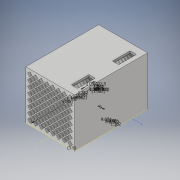
# Autodesk Inventor part: Double Holder V1
Saved by Autodesk Inventor 2019 (Build 230136000, 136)
## iProperties
Created: 2018-11-20
Part Number: Double Holder V1
Material: Generic
Document SubType Name: Modeling
Designer: Ashley
Density: 1 g/cm^3
Appearance: Default
Author: Ashley
Autodesk Inventor part; units mm, degrees
(part 1 of 2)
ref_plane "YZ Plane" through (0, 0, 0) normal (1, 0, 0) x (0, 1, 0)
ref_plane "XZ Plane" through (0, 0, 0) normal (0, 1, 0) x (-1, 0, 0)
ref_plane "XY Plane" through (0, 0, 0) normal (0, 0, 1) x (1, 0, 0)
sketch "Main Body Sketch" plane through (0, 0, 0) normal (0, 1, 0) x (-1, 0, 0)
  line L0 (-38.5, 7.5) -> (38.5, 7.5)
  line L1 (38.5, 7.5) -> (38.5, 57.5)
  line L2 (38.5, 57.5) -> (-38.5, 57.5)
  line L3 (-38.5, 57.5) -> (-38.5, 7.5)
  line L4 (0, 222.8068) -> (0, -187.3036) construction
  line L5 (63.0186, 0) -> (-52.8672, 0) construction
  line L6 (-38.5, -7.5) -> (38.5, -7.5)
  line L7 (38.5, -7.5) -> (38.5, -57.5)
  line L8 (38.5, -57.5) -> (-38.5, -57.5)
  line L9 (-38.5, -57.5) -> (-38.5, -7.5)
  line L10 (0, -222.8068) -> (0, 187.3036) construction
  point P0 (0, 0)
  dimension "d2" = 50
  dimension "d3" = 77
  dimension "d4" = 38.5
  dimension "d5" = 38.5
  dimension "d6" = 7.5
  constraints: 22 end point, 6 symmetric about line, 3 horizontal, 2 parallel, 2 vertical, 1 perpendicular
  measures "d2" distance of L0.end L1.end
  measures "d3" distance of L1.end L2.end
  measures "d4" distance between parallel lines of L4 L1
  measures "d5" distance between parallel lines of L3 L4
  measures "d6" distance between parallel lines of L5 L0
extrude "Main Body Extrusion" add sketch "Main Body Sketch" along normal blind 77
sketch "Main Compartments Sketch" plane through (-38.5, 0, 7.5) normal (-1, 0, 0) x (0, 0, 1)
  line L0 (0, 0) -> (50, 0) construction
  line L1 (-61.5, 3.5) -> (-18.5, 3.5)
  line L2 (-18.5, 3.5) -> (-18.5, 73.5)
  line L3 (-18.5, 73.5) -> (-61.5, 73.5)
  line L4 (-61.5, 73.5) -> (-61.5, 3.5)
  line L5 (-65, 77) -> (-15, 77) construction
  line L6 (-15, 0) -> (-65, 0) construction
  line L7 (-65, 0) -> (-65, 77) construction
  line L8 (-15, 0) -> (-15, 77) construction
  line L9 (-7.5, -40.8537) -> (-7.5, 113.2873) construction
  line L10 (46.5, 3.5) -> (3.5, 3.5)
  line L11 (3.5, 3.5) -> (3.5, 73.5)
  line L12 (3.5, 73.5) -> (46.5, 73.5)
  line L13 (46.5, 73.5) -> (46.5, 3.5)
  line L14 (50, 77) -> (0, 77) construction
  line L15 (0, 0) -> (50, 0) construction
  line L16 (50, 0) -> (50, 77) construction
  line L17 (0, 0) -> (0, 77) construction
  point P0 (-7.5, 0)
  dimension "d10" = 70
  dimension "d11" = 3.5
  dimension "d12" = 3.5
  dimension "d13" = 43
  dimension "d14" = 3.5
  dimension "d15" = 3.5
  dimension "d16" = 3.5
  dimension "d17" = 3.5
  constraints: 26 end point, 4 symmetric about line, 2 parallel, 2 vertical, 1 horizontal, 1 perpendicular
  measures "d10" distance of L3.end L1.start
  measures "d11" distance between parallel lines of L5 L3
  measures "d12" distance between parallel lines of L6 L1
  measures "d13" distance between parallel lines of L2 L4
  measures "d14" distance between parallel lines of L7 L4
  measures "d15" distance between parallel lines of L8 L2
  measures "d16" distance between parallel lines of L17 L11
  measures "d17" distance between parallel lines of L0 L10
extrude "Main Compartments Extrusion" cut sketch "Main Compartments Sketch" against normal blind 73.5
sketch "Tape Measure Hole Sketch" plane through (0, 77, 0) normal (0, 1, 0) x (1, 0, 0)
  line L0 (38.5, -57.5) -> (38.5, 57.5) construction
  line L1 (22, -46.5) -> (32, -46.5)
  line L2 (32, -46.5) -> (32, -18.5)
  line L3 (32, -18.5) -> (22, -18.5)
  line L4 (22, -18.5) -> (22, -46.5)
  line L5 (-52.0293, 0) -> (49.471, 0) construction
  line L6 (-38.5, -11) -> (35, -11) construction
  line L7 (4.7749, -11) -> (35, -11) construction
  line L8 (-38.5, -54) -> (35, -54) construction
  line L9 (22, 46.5) -> (32, 46.5)
  line L10 (32, 46.5) -> (32, 18.5)
  line L11 (32, 18.5) -> (22, 18.5)
  line L12 (22, 18.5) -> (22, 46.5)
  line L13 (-38.5, -54) -> (35, -54) construction
  line L14 (35, -54) -> (35, -11) construction
  point P0 (0, 0)
  dimension "d26" = 10
  dimension "d27" = 6.5
  dimension "d28" = 28
  dimension "d32" = 11
  dimension "d33" = 43
  dimension "d34" = 7.5
  dimension "d35" = 7.5
  dimension "d38" = 3.5
  dimension "d39" = 3
  constraints: 22 end point, 4 horizontal, 4 symmetric about line, 3 parallel, 1 collinear, 1 perpendicular, 1 point on line, 1 vertical
  measures "d26" distance of L2.end L3.end
  measures "d27" distance between parallel lines of L0 L2
  measures "d28" distance of L3.end L1.start
  measures "d32" distance between parallel lines of L5 L6
  measures "d33" distance between parallel lines of L6 L8
  measures "d34" distance between parallel lines of L8 L1
  measures "d35" distance between parallel lines of L3 L7
  measures "d38" distance between parallel lines of L0 L14
  measures "d39" distance between parallel lines of L14 L2
extrude "Tape Measure Holes Cut" cut sketch "Tape Measure Hole Sketch" against normal up to surface (3.5 mm away)
fillet "Tape Measure Holes Softening" radius 1 8 edges at (22, 75.25, 46.5) (32, 75.25, 46.5) (22, 75.25, 18.5) (32, 75.25, 18.5) (32, 75.25, -46.5) (22, 75.25, -46.5) (22, 75.25, -18.5) (32, 75.25, -18.5)
sketch "Center Sketch" plane through (38.5, 0, 7.5) normal (0, 0, -1) x (-1, 0, 0)
  line L0 (77, 77) -> (0, 77)
  line L1 (0, 77) -> (0, 0)
  line L2 (0, 0) -> (77, 0)
  line L3 (77, 0) -> (77, 77)
  point P0 (38.5, 0)
  constraints: 8 end point, 2 parallel, 1 horizontal, 1 perpendicular
extrude "Center Extrusion" add sketch "Center Sketch" along normal up to surface (15 mm away)
sketch "Swiss Holes Sketch" plane through (38.5, 0, -57.5) normal (0, 0, -1) x (-1, 0, 0)
  line L0 (0, 77) -> (77, 77) construction
  line L1 (77, 73.5) -> (3.5, 73.5) construction
  line L2 (3.5, 73.5) -> (3.5, 3.5) construction
  line L3 (77, 73.5) -> (3.5, 73.5) construction
  line L4 (3.5, 73.5) -> (3.5, 3.5) construction
  line L5 (3.5, 3.5) -> (77, 3.5) construction
  line L6 (66.9969, 69.9645) -> (70.5325, 73.5)
  line L7 (70.5325, 73.5) -> (74.068, 69.9645)
  line L8 (74.068, 69.9645) -> (70.5325, 66.4289)
  line L9 (70.5325, 66.4289) -> (66.9969, 69.9645)
  line L10 (77, 0) -> (77, 77) construction
  line L11 (61.4615, 66.4289) -> (57.9259, 69.9645)
  line L12 (61.4615, 73.5) -> (64.997, 69.9645)
  line L13 (64.997, 69.9645) -> (61.4615, 66.4289)
  line L14 (67.929, 73.5) -> (-5.571, 73.5) construction
  line L15 (57.9259, 69.9645) -> (61.4615, 73.5)
  line L16 (52.3905, 66.4289) -> (48.8549, 69.9645)
  line L17 (52.3905, 73.5) -> (55.926, 69.9645)
  line L18 (55.926, 69.9645) -> (52.3905, 66.4289)
  line L19 (58.858, 73.5) -> (-14.642, 73.5) construction
  line L20 (48.8549, 69.9645) -> (52.3905, 73.5)
  line L21 (43.3195, 66.4289) -> (39.7839, 69.9645)
  line L22 (43.3195, 73.5) -> (46.855, 69.9645)
  line L23 (46.855, 69.9645) -> (43.3195, 66.4289)
  line L24 (49.787, 73.5) -> (-23.713, 73.5) construction
  line L25 (39.7839, 69.9645) -> (43.3195, 73.5)
  line L26 (34.2485, 66.4289) -> (30.7129, 69.9645)
  line L27 (34.2485, 73.5) -> (37.784, 69.9645)
  line L28 (37.784, 69.9645) -> (34.2485, 66.4289)
  line L29 (40.716, 73.5) -> (-32.784, 73.5) construction
  line L30 (30.7129, 69.9645) -> (34.2485, 73.5)
  line L31 (25.1775, 66.4289) -> (21.6419, 69.9645)
  line L32 (25.1775, 73.5) -> (28.713, 69.9645)
  line L33 (28.713, 69.9645) -> (25.1775, 66.4289)
  line L34 (31.645, 73.5) -> (-41.855, 73.5) construction
  line L35 (21.6419, 69.9645) -> (25.1775, 73.5)
  line L36 (16.1065, 66.4289) -> (12.5709, 69.9645)
  line L37 (16.1065, 73.5) -> (19.642, 69.9645)
  line L38 (19.642, 69.9645) -> (16.1065, 66.4289)
  line L39 (22.574, 73.5) -> (-50.926, 73.5) construction
  line L40 (12.5709, 69.9645) -> (16.1065, 73.5)
  line L41 (7.0355, 66.4289) -> (3.4999, 69.9645)
  line L42 (7.0355, 73.5) -> (10.571, 69.9645)
  line L43 (10.571, 69.9645) -> (7.0355, 66.4289)
  line L44 (13.503, 73.5) -> (-59.997, 73.5) construction
  line L45 (3.4999, 69.9645) -> (7.0355, 73.5)
  line L46 (70.5325, 57.4489) -> (66.9969, 60.9845)
  line L47 (70.5325, 64.52) -> (74.068, 60.9845)
  line L48 (74.068, 60.9845) -> (70.5325, 57.4489)
  line L49 (77, 64.52) -> (3.5, 64.52) construction
  line L50 (66.9969, 60.9845) -> (70.5325, 64.52)
  line L51 (61.4615, 57.4489) -> (57.9259, 60.9845)
  line L52 (61.4615, 64.52) -> (64.997, 60.9845)
  line L53 (64.997, 60.9845) -> (61.4615, 57.4489)
  line L54 (67.929, 64.52) -> (-5.571, 64.52) construction
  line L55 (57.9259, 60.9845) -> (61.4615, 64.52)
  line L56 (52.3905, 57.4489) -> (48.8549, 60.9845)
  line L57 (52.3905, 64.52) -> (55.926, 60.9845)
  line L58 (55.926, 60.9845) -> (52.3905, 57.4489)
  line L59 (58.858, 64.52) -> (-14.642, 64.52) construction
  line L60 (48.8549, 60.9845) -> (52.3905, 64.52)
  line L61 (43.3195, 57.4489) -> (39.7839, 60.9845)
  line L62 (43.3195, 64.52) -> (46.855, 60.9845)
  line L63 (46.855, 60.9845) -> (43.3195, 57.4489)
  line L64 (49.787, 64.52) -> (-23.713, 64.52) construction
  line L65 (39.7839, 60.9845) -> (43.3195, 64.52)
  line L66 (34.2485, 57.4489) -> (30.7129, 60.9845)
  line L67 (34.2485, 64.52) -> (37.784, 60.9845)
  line L68 (37.784, 60.9845) -> (34.2485, 57.4489)
  line L69 (40.716, 64.52) -> (-32.784, 64.52) construction
  line L70 (30.7129, 60.9845) -> (34.2485, 64.52)
  line L71 (25.1775, 57.4489) -> (21.6419, 60.9845)
  line L72 (25.1775, 64.52) -> (28.713, 60.9845)
  line L73 (28.713, 60.9845) -> (25.1775, 57.4489)
  line L74 (31.645, 64.52) -> (-41.855, 64.52) construction
  line L75 (21.6419, 60.9845) -> (25.1775, 64.52)
  line L76 (16.1065, 57.4489) -> (12.5709, 60.9845)
  line L77 (16.1065, 64.52) -> (19.642, 60.9845)
  line L78 (19.642, 60.9845) -> (16.1065, 57.4489)
  line L79 (22.574, 64.52) -> (-50.926, 64.52) construction
  line L80 (12.5709, 60.9845) -> (16.1065, 64.52)
  line L81 (7.0355, 57.4489) -> (3.4999, 60.9845)
  line L82 (7.0355, 64.52) -> (10.571, 60.9845)
  line L83 (10.571, 60.9845) -> (7.0355, 57.4489)
  line L84 (13.503, 64.52) -> (-59.997, 64.52) construction
  line L85 (3.4999, 60.9845) -> (7.0355, 64.52)
  line L86 (70.5325, 48.4689) -> (66.9969, 52.0045)
  line L87 (70.5325, 55.54) -> (74.068, 52.0045)
  line L88 (74.068, 52.0045) -> (70.5325, 48.4689)
  line L89 (77, 55.54) -> (3.5, 55.54) construction
  line L90 (66.9969, 52.0045) -> (70.5325, 55.54)
  line L91 (61.4615, 48.4689) -> (57.9259, 52.0045)
  line L92 (61.4615, 55.54) -> (64.997, 52.0045)
  line L93 (64.997, 52.0045) -> (61.4615, 48.4689)
  line L94 (67.929, 55.54) -> (-5.571, 55.54) construction
  line L95 (57.9259, 52.0045) -> (61.4615, 55.54)
  line L96 (52.3905, 48.4689) -> (48.8549, 52.0045)
  line L97 (52.3905, 55.54) -> (55.926, 52.0045)
  line L98 (55.926, 52.0045) -> (52.3905, 48.4689)
  line L99 (58.858, 55.54) -> (-14.642, 55.54) construction
  line L100 (48.8549, 52.0045) -> (52.3905, 55.54)
  line L101 (43.3195, 48.4689) -> (39.7839, 52.0045)
  line L102 (43.3195, 55.54) -> (46.855, 52.0045)
  line L103 (46.855, 52.0045) -> (43.3195, 48.4689)
  line L104 (49.787, 55.54) -> (-23.713, 55.54) construction
  line L105 (39.7839, 52.0045) -> (43.3195, 55.54)
  line L106 (34.2485, 48.4689) -> (30.7129, 52.0045)
  line L107 (34.2485, 55.54) -> (37.784, 52.0045)
  line L108 (37.784, 52.0045) -> (34.2485, 48.4689)
  line L109 (40.716, 55.54) -> (-32.784, 55.54) construction
  line L110 (30.7129, 52.0045) -> (34.2485, 55.54)
  line L111 (25.1775, 48.4689) -> (21.6419, 52.0045)
  line L112 (25.1775, 55.54) -> (28.713, 52.0045)
  line L113 (28.713, 52.0045) -> (25.1775, 48.4689)
  line L114 (31.645, 55.54) -> (-41.855, 55.54) construction
  line L115 (21.6419, 52.0045) -> (25.1775, 55.54)
  line L116 (16.1065, 48.4689) -> (12.5709, 52.0045)
  line L117 (16.1065, 55.54) -> (19.642, 52.0045)
  line L118 (19.642, 52.0045) -> (16.1065, 48.4689)
  line L119 (22.574, 55.54) -> (-50.926, 55.54) construction
  line L120 (12.5709, 52.0045) -> (16.1065, 55.54)
  line L121 (7.0355, 48.4689) -> (3.4999, 52.0045)
  line L122 (7.0355, 55.54) -> (10.571, 52.0045)
  line L123 (10.571, 52.0045) -> (7.0355, 48.4689)
  line L124 (13.503, 55.54) -> (-59.997, 55.54) construction
  line L125 (3.4999, 52.0045) -> (7.0355, 55.54)
  line L126 (70.5325, 39.4889) -> (66.9969, 43.0245)
  line L127 (70.5325, 46.56) -> (74.068, 43.0245)
  line L128 (74.068, 43.0245) -> (70.5325, 39.4889)
  line L129 (77, 46.56) -> (3.5, 46.56) construction
  line L130 (66.9969, 43.0245) -> (70.5325, 46.56)
  line L131 (61.4615, 39.4889) -> (57.9259, 43.0245)
  line L132 (61.4615, 46.56) -> (64.997, 43.0245)
  line L133 (64.997, 43.0245) -> (61.4615, 39.4889)
  line L134 (67.929, 46.56) -> (-5.571, 46.56) construction
  line L135 (57.9259, 43.0245) -> (61.4615, 46.56)
  line L136 (52.3905, 39.4889) -> (48.8549, 43.0245)
  line L137 (52.3905, 46.56) -> (55.926, 43.0245)
  line L138 (55.926, 43.0245) -> (52.3905, 39.4889)
  line L139 (58.858, 46.56) -> (-14.642, 46.56) construction
  line L140 (48.8549, 43.0245) -> (52.3905, 46.56)
  line L141 (43.3195, 39.4889) -> (39.7839, 43.0245)
  line L142 (43.3195, 46.56) -> (46.855, 43.0245)
  line L143 (46.855, 43.0245) -> (43.3195, 39.4889)
  line L144 (49.787, 46.56) -> (-23.713, 46.56) construction
  line L145 (39.7839, 43.0245) -> (43.3195, 46.56)
  line L146 (34.2485, 39.4889) -> (30.7129, 43.0245)
  line L147 (34.2485, 46.56) -> (37.784, 43.0245)
  line L148 (37.784, 43.0245) -> (34.2485, 39.4889)
  line L149 (40.716, 46.56) -> (-32.784, 46.56) construction
  line L150 (30.7129, 43.0245) -> (34.2485, 46.56)
  line L151 (25.1775, 39.4889) -> (21.6419, 43.0245)
  line L152 (25.1775, 46.56) -> (28.713, 43.0245)
  line L153 (28.713, 43.0245) -> (25.1775, 39.4889)
  line L154 (31.645, 46.56) -> (-41.855, 46.56) construction
  line L155 (21.6419, 43.0245) -> (25.1775, 46.56)
  line L156 (16.1065, 39.4889) -> (12.5709, 43.0245)
  line L157 (16.1065, 46.56) -> (19.642, 43.0245)
  line L158 (19.642, 43.0245) -> (16.1065, 39.4889)
  line L159 (22.574, 46.56) -> (-50.926, 46.56) construction
  line L160 (12.5709, 43.0245) -> (16.1065, 46.56)
  line L161 (7.0355, 39.4889) -> (3.4999, 43.0245)
  line L162 (7.0355, 46.56) -> (10.571, 43.0245)
  line L163 (10.571, 43.0245) -> (7.0355, 39.4889)
  line L164 (13.503, 46.56) -> (-59.997, 46.56) construction
  line L165 (3.4999, 43.0245) -> (7.0355, 46.56)
  line L166 (70.5325, 30.5089) -> (66.9969, 34.0445)
  line L167 (70.5325, 37.58) -> (74.068, 34.0445)
  line L168 (74.068, 34.0445) -> (70.5325, 30.5089)
  line L169 (77, 37.58) -> (3.5, 37.58) construction
  line L170 (66.9969, 34.0445) -> (70.5325, 37.58)
  line L171 (61.4615, 30.5089) -> (57.9259, 34.0445)
  line L172 (61.4615, 37.58) -> (64.997, 34.0445)
  line L173 (64.997, 34.0445) -> (61.4615, 30.5089)
  line L174 (67.929, 37.58) -> (-5.571, 37.58) construction
  line L175 (57.9259, 34.0445) -> (61.4615, 37.58)
  line L176 (52.3905, 30.5089) -> (48.8549, 34.0445)
  line L177 (52.3905, 37.58) -> (55.926, 34.0445)
  line L178 (55.926, 34.0445) -> (52.3905, 30.5089)
  line L179 (58.858, 37.58) -> (-14.642, 37.58) construction
  line L180 (48.8549, 34.0445) -> (52.3905, 37.58)
  line L181 (43.3195, 30.5089) -> (39.7839, 34.0445)
  line L182 (43.3195, 37.58) -> (46.855, 34.0445)
  line L183 (46.855, 34.0445) -> (43.3195, 30.5089)
  line L184 (49.787, 37.58) -> (-23.713, 37.58) construction
  line L185 (39.7839, 34.0445) -> (43.3195, 37.58)
  line L186 (34.2485, 30.5089) -> (30.7129, 34.0445)
  line L187 (34.2485, 37.58) -> (37.784, 34.0445)
  line L188 (37.784, 34.0445) -> (34.2485, 30.5089)
  line L189 (40.716, 37.58) -> (-32.784, 37.58) construction
  line L190 (30.7129, 34.0445) -> (34.2485, 37.58)
  line L191 (25.1775, 30.5089) -> (21.6419, 34.0445)
  line L192 (25.1775, 37.58) -> (28.713, 34.0445)
  line L193 (28.713, 34.0445) -> (25.1775, 30.5089)
  line L194 (31.645, 37.58) -> (-41.855, 37.58) construction
  line L195 (21.6419, 34.0445) -> (25.1775, 37.58)
  line L196 (16.1065, 30.5089) -> (12.5709, 34.0445)
  line L197 (16.1065, 37.58) -> (19.642, 34.0445)
  line L198 (19.642, 34.0445) -> (16.1065, 30.5089)
  line L199 (22.574, 37.58) -> (-50.926, 37.58) construction
  line L200 (12.5709, 34.0445) -> (16.1065, 37.58)
  line L201 (7.0355, 30.5089) -> (3.4999, 34.0445)
  line L202 (7.0355, 37.58) -> (10.571, 34.0445)
  line L203 (10.571, 34.0445) -> (7.0355, 30.5089)
  line L204 (13.503, 37.58) -> (-59.997, 37.58) construction
  line L205 (3.4999, 34.0445) -> (7.0355, 37.58)
  line L206 (70.5325, 21.5289) -> (66.9969, 25.0645)
  line L207 (70.5325, 28.6) -> (74.068, 25.0645)
  line L208 (74.068, 25.0645) -> (70.5325, 21.5289)
  line L209 (77, 28.6) -> (3.5, 28.6) construction
  line L210 (66.9969, 25.0645) -> (70.5325, 28.6)
  line L211 (61.4615, 21.5289) -> (57.9259, 25.0645)
  line L212 (61.4615, 28.6) -> (64.997, 25.0645)
  line L213 (64.997, 25.0645) -> (61.4615, 21.5289)
  line L214 (67.929, 28.6) -> (-5.571, 28.6) construction
  line L215 (57.9259, 25.0645) -> (61.4615, 28.6)
  line L216 (52.3905, 21.5289) -> (48.8549, 25.0645)
  line L217 (52.3905, 28.6) -> (55.926, 25.0645)
  line L218 (55.926, 25.0645) -> (52.3905, 21.5289)
  line L219 (58.858, 28.6) -> (-14.642, 28.6) construction
  line L220 (48.8549, 25.0645) -> (52.3905, 28.6)
  line L221 (43.3195, 21.5289) -> (39.7839, 25.0645)
  line L222 (43.3195, 28.6) -> (46.855, 25.0645)
  line L223 (46.855, 25.0645) -> (43.3195, 21.5289)
  line L224 (49.787, 28.6) -> (-23.713, 28.6) construction
  line L225 (39.7839, 25.0645) -> (43.3195, 28.6)
  line L226 (34.2485, 21.5289) -> (30.7129, 25.0645)
  line L227 (34.2485, 28.6) -> (37.784, 25.0645)
  line L228 (37.784, 25.0645) -> (34.2485, 21.5289)
  line L229 (40.716, 28.6) -> (-32.784, 28.6) construction
  line L230 (30.7129, 25.0645) -> (34.2485, 28.6)
  line L231 (25.1775, 21.5289) -> (21.6419, 25.0645)
  line L232 (25.1775, 28.6) -> (28.713, 25.0645)
  line L233 (28.713, 25.0645) -> (25.1775, 21.5289)
  line L234 (31.645, 28.6) -> (-41.855, 28.6) construction
  line L235 (21.6419, 25.0645) -> (25.1775, 28.6)
  line L236 (16.1065, 21.5289) -> (12.5709, 25.0645)
  line L237 (16.1065, 28.6) -> (19.642, 25.0645)
  line L238 (19.642, 25.0645) -> (16.1065, 21.5289)
  line L239 (22.574, 28.6) -> (-50.926, 28.6) construction
  line L240 (12.5709, 25.0645) -> (16.1065, 28.6)
  line L241 (7.0355, 21.5289) -> (3.4999, 25.0645)
  line L242 (7.0355, 28.6) -> (10.571, 25.0645)
  line L243 (10.571, 25.0645) -> (7.0355, 21.5289)
  line L244 (13.503, 28.6) -> (-59.997, 28.6) construction
  line L245 (3.4999, 25.0645) -> (7.0355, 28.6)
  line L246 (70.5325, 12.5489) -> (66.9969, 16.0845)
  line L247 (70.5325, 19.62) -> (74.068, 16.0845)
  line L248 (74.068, 16.0845) -> (70.5325, 12.5489)
  line L249 (77, 19.62) -> (3.5, 19.62) construction
  line L250 (66.9969, 16.0845) -> (70.5325, 19.62)
  line L251 (61.4615, 12.5489) -> (57.9259, 16.0845)
  line L252 (61.4615, 19.62) -> (64.997, 16.0845)
  line L253 (64.997, 16.0845) -> (61.4615, 12.5489)
  line L254 (67.929, 19.62) -> (-5.571, 19.62) construction
  line L255 (57.9259, 16.0845) -> (61.4615, 19.62)
  line L256 (52.3905, 12.5489) -> (48.8549, 16.0845)
  line L257 (52.3905, 19.62) -> (55.926, 16.0845)
  line L258 (55.926, 16.0845) -> (52.3905, 12.5489)
  line L259 (58.858, 19.62) -> (-14.642, 19.62) construction
  line L260 (48.8549, 16.0845) -> (52.3905, 19.62)
  line L261 (43.3195, 12.5489) -> (39.7839, 16.0845)
  line L262 (43.3195, 19.62) -> (46.855, 16.0845)
  line L263 (46.855, 16.0845) -> (43.3195, 12.5489)
  line L264 (49.787, 19.62) -> (-23.713, 19.62) construction
  line L265 (39.7839, 16.0845) -> (43.3195, 19.62)
  line L266 (34.2485, 12.5489) -> (30.7129, 16.0845)
  line L267 (34.2485, 19.62) -> (37.784, 16.0845)
  line L268 (37.784, 16.0845) -> (34.2485, 12.5489)
  line L269 (40.716, 19.62) -> (-32.784, 19.62) construction
  line L270 (30.7129, 16.0845) -> (34.2485, 19.62)
  line L271 (25.1775, 12.5489) -> (21.6419, 16.0845)
  line L272 (25.1775, 19.62) -> (28.713, 16.0845)
  line L273 (28.713, 16.0845) -> (25.1775, 12.5489)
  line L274 (31.645, 19.62) -> (-41.855, 19.62) construction
  line L275 (21.6419, 16.0845) -> (25.1775, 19.62)
  line L276 (16.1065, 12.5489) -> (12.5709, 16.0845)
  line L277 (16.1065, 19.62) -> (19.642, 16.0845)
  line L278 (19.642, 16.0845) -> (16.1065, 12.5489)
  line L279 (22.574, 19.62) -> (-50.926, 19.62) construction
  line L280 (12.5709, 16.0845) -> (16.1065, 19.62)
  line L281 (7.0355, 12.5489) -> (3.4999, 16.0845)
  line L282 (7.0355, 19.62) -> (10.571, 16.0845)
  line L283 (10.571, 16.0845) -> (7.0355, 12.5489)
  line L284 (13.503, 19.62) -> (-59.997, 19.62) construction
  line L285 (3.4999, 16.0845) -> (7.0355, 19.62)
  line L286 (70.5325, 3.5689) -> (66.9969, 7.1045)
  line L287 (70.5325, 10.64) -> (74.068, 7.1045)
  line L288 (74.068, 7.1045) -> (70.5325, 3.5689)
  line L289 (77, 10.64) -> (3.5, 10.64) construction
  line L290 (66.9969, 7.1045) -> (70.5325, 10.64)
  line L291 (61.4615, 3.5689) -> (57.9259, 7.1045)
  line L292 (61.4615, 10.64) -> (64.997, 7.1045)
  line L293 (64.997, 7.1045) -> (61.4615, 3.5689)
  line L294 (67.929, 10.64) -> (-5.571, 10.64) construction
  line L295 (57.9259, 7.1045) -> (61.4615, 10.64)
  line L296 (52.3905, 3.5689) -> (48.8549, 7.1045)
  line L297 (52.3905, 10.64) -> (55.926, 7.1045)
  line L298 (55.926, 7.1045) -> (52.3905, 3.5689)
  line L299 (58.858, 10.64) -> (-14.642, 10.64) construction
  line L300 (48.8549, 7.1045) -> (52.3905, 10.64)
  line L301 (43.3195, 3.5689) -> (39.7839, 7.1045)
  line L302 (43.3195, 10.64) -> (46.855, 7.1045)
  line L303 (46.855, 7.1045) -> (43.3195, 3.5689)
  line L304 (49.787, 10.64) -> (-23.713, 10.64) construction
  line L305 (39.7839, 7.1045) -> (43.3195, 10.64)
  line L306 (34.2485, 3.5689) -> (30.7129, 7.1045)
  line L307 (34.2485, 10.64) -> (37.784, 7.1045)
  line L308 (37.784, 7.1045) -> (34.2485, 3.5689)
  line L309 (40.716, 10.64) -> (-32.784, 10.64) construction
  line L310 (30.7129, 7.1045) -> (34.2485, 10.64)
  line L311 (25.1775, 3.5689) -> (21.6419, 7.1045)
  line L312 (25.1775, 10.64) -> (28.713, 7.1045)
  line L313 (28.713, 7.1045) -> (25.1775, 3.5689)
  line L314 (31.645, 10.64) -> (-41.855, 10.64) construction
  line L315 (21.6419, 7.1045) -> (25.1775, 10.64)
  line L316 (16.1065, 3.5689) -> (12.5709, 7.1045)
  line L317 (16.1065, 10.64) -> (19.642, 7.1045)
  line L318 (19.642, 7.1045) -> (16.1065, 3.5689)
  line L319 (22.574, 10.64) -> (-50.926, 10.64) construction
  line L320 (12.5709, 7.1045) -> (16.1065, 10.64)
  line L321 (7.0355, 3.5689) -> (3.4999, 7.1045)
  line L322 (7.0355, 10.64) -> (10.571, 7.1045)
  line L323 (10.571, 7.1045) -> (7.0355, 3.5689)
  line L324 (13.503, 10.64) -> (-59.997, 10.64) construction
  line L325 (3.4999, 7.1045) -> (7.0355, 10.64)
  line L326 (65.9973, 61.9389) -> (69.5328, 65.4745)
  line L327 (69.5328, 65.4745) -> (65.9973, 69.01)
  line L328 (65.9973, 69.01) -> (62.4618, 65.4745)
  line L329 (62.4618, 65.4745) -> (65.9973, 61.9389)
  line L330 (58.858, 64.52) -> (-14.642, 64.52) construction
  line L331 (67.929, 64.52) -> (-5.571, 64.52) construction
  line L332 (53.3908, 65.4745) -> (56.9263, 61.9389)
  line L333 (56.9263, 69.01) -> (53.3908, 65.4745)
  line L334 (56.9263, 61.9389) -> (60.4618, 65.4745)
  line L335 (60.4618, 65.4745) -> (56.9263, 69.01)
  line L336 (49.787, 64.52) -> (-23.713, 64.52) construction
  line L337 (58.858, 64.52) -> (-14.642, 64.52) construction
  line L338 (44.3198, 65.4745) -> (47.8553, 61.9389)
  line L339 (47.8553, 69.01) -> (44.3198, 65.4745)
  line L340 (47.8553, 61.9389) -> (51.3908, 65.4745)
  line L341 (51.3908, 65.4745) -> (47.8553, 69.01)
  line L342 (40.716, 64.52) -> (-32.784, 64.52) construction
  line L343 (49.787, 64.52) -> (-23.713, 64.52) construction
  line L344 (35.2488, 65.4745) -> (38.7843, 61.9389)
  line L345 (38.7843, 69.01) -> (35.2488, 65.4745)
  line L346 (38.7843, 61.9389) -> (42.3198, 65.4745)
  line L347 (42.3198, 65.4745) -> (38.7843, 69.01)
  line L348 (31.645, 64.52) -> (-41.855, 64.52) construction
  line L349 (40.716, 64.52) -> (-32.784, 64.52) construction
  line L350 (26.1778, 65.4745) -> (29.7133, 61.9389)
  line L351 (29.7133, 69.01) -> (26.1778, 65.4745)
  line L352 (29.7133, 61.9389) -> (33.2488, 65.4745)
  line L353 (33.2488, 65.4745) -> (29.7133, 69.01)
  line L354 (22.574, 64.52) -> (-50.926, 64.52) construction
  line L355 (31.645, 64.52) -> (-41.855, 64.52) construction
  line L356 (17.1068, 65.4745) -> (20.6423, 61.9389)
  line L357 (20.6423, 69.01) -> (17.1068, 65.4745)
  line L358 (20.6423, 61.9389) -> (24.1778, 65.4745)
  line L359 (24.1778, 65.4745) -> (20.6423, 69.01)
  line L360 (13.503, 64.52) -> (-59.997, 64.52) construction
  line L361 (22.574, 64.52) -> (-50.926, 64.52) construction
  line L362 (8.0358, 65.4745) -> (11.5713, 61.9389)
  line L363 (11.5713, 69.01) -> (8.0358, 65.4745)
  line L364 (11.5713, 61.9389) -> (15.1068, 65.4745)
  line L365 (15.1068, 65.4745) -> (11.5713, 69.01)
  line L366 (67.929, 55.54) -> (-5.571, 55.54) construction
  line L367 (77, 55.54) -> (3.5, 55.54) construction
  line L368 (62.4618, 56.4945) -> (65.9973, 52.9589)
  line L369 (65.9973, 60.03) -> (62.4618, 56.4945)
  line L370 (65.9973, 52.9589) -> (69.5328, 56.4945)
  line L371 (69.5328, 56.4945) -> (65.9973, 60.03)
  line L372 (58.858, 55.54) -> (-14.642, 55.54) construction
  line L373 (67.929, 55.54) -> (-5.571, 55.54) construction
  line L374 (53.3908, 56.4945) -> (56.9263, 52.9589)
  line L375 (56.9263, 60.03) -> (53.3908, 56.4945)
  line L376 (56.9263, 52.9589) -> (60.4618, 56.4945)
  line L377 (60.4618, 56.4945) -> (56.9263, 60.03)
  line L378 (49.787, 55.54) -> (-23.713, 55.54) construction
  line L379 (58.858, 55.54) -> (-14.642, 55.54) construction
  line L380 (44.3198, 56.4945) -> (47.8553, 52.9589)
  line L381 (47.8553, 60.03) -> (44.3198, 56.4945)
  line L382 (47.8553, 52.9589) -> (51.3908, 56.4945)
  line L383 (51.3908, 56.4945) -> (47.8553, 60.03)
  line L384 (40.716, 55.54) -> (-32.784, 55.54) construction
  line L385 (49.787, 55.54) -> (-23.713, 55.54) construction
  line L386 (35.2488, 56.4945) -> (38.7843, 52.9589)
  line L387 (38.7843, 60.03) -> (35.2488, 56.4945)
  line L388 (38.7843, 52.9589) -> (42.3198, 56.4945)
  line L389 (42.3198, 56.4945) -> (38.7843, 60.03)
  line L390 (31.645, 55.54) -> (-41.855, 55.54) construction
  line L391 (40.716, 55.54) -> (-32.784, 55.54) construction
  line L392 (26.1778, 56.4945) -> (29.7133, 52.9589)
  line L393 (29.7133, 60.03) -> (26.1778, 56.4945)
  line L394 (29.7133, 52.9589) -> (33.2488, 56.4945)
  line L395 (33.2488, 56.4945) -> (29.7133, 60.03)
  line L396 (22.574, 55.54) -> (-50.926, 55.54) construction
  line L397 (31.645, 55.54) -> (-41.855, 55.54) construction
  line L398 (17.1068, 56.4945) -> (20.6423, 52.9589)
  line L399 (20.6423, 60.03) -> (17.1068, 56.4945)
  line L400 (20.6423, 52.9589) -> (24.1778, 56.4945)
  line L401 (24.1778, 56.4945) -> (20.6423, 60.03)
  line L402 (13.503, 55.54) -> (-59.997, 55.54) construction
  line L403 (22.574, 55.54) -> (-50.926, 55.54) construction
  line L404 (8.0358, 56.4945) -> (11.5713, 52.9589)
  line L405 (11.5713, 60.03) -> (8.0358, 56.4945)
  line L406 (11.5713, 52.9589) -> (15.1068, 56.4945)
  line L407 (15.1068, 56.4945) -> (11.5713, 60.03)
  line L408 (67.929, 46.56) -> (-5.571, 46.56) construction
  line L409 (77, 46.56) -> (3.5, 46.56) construction
  line L410 (62.4618, 47.5145) -> (65.9973, 43.9789)
  line L411 (65.9973, 51.05) -> (62.4618, 47.5145)
  line L412 (65.9973, 43.9789) -> (69.5328, 47.5145)
  line L413 (69.5328, 47.5145) -> (65.9973, 51.05)
  line L414 (58.858, 46.56) -> (-14.642, 46.56) construction
  line L415 (67.929, 46.56) -> (-5.571, 46.56) construction
  line L416 (53.3908, 47.5145) -> (56.9263, 43.9789)
  line L417 (56.9263, 51.05) -> (53.3908, 47.5145)
  line L418 (56.9263, 43.9789) -> (60.4618, 47.5145)
  line L419 (60.4618, 47.5145) -> (56.9263, 51.05)
  line L420 (49.787, 46.56) -> (-23.713, 46.56) construction
  line L421 (58.858, 46.56) -> (-14.642, 46.56) construction
  line L422 (44.3198, 47.5145) -> (47.8553, 43.9789)
  line L423 (47.8553, 51.05) -> (44.3198, 47.5145)
  line L424 (47.8553, 43.9789) -> (51.3908, 47.5145)
  line L425 (51.3908, 47.5145) -> (47.8553, 51.05)
  line L426 (40.716, 46.56) -> (-32.784, 46.56) construction
  line L427 (49.787, 46.56) -> (-23.713, 46.56) construction
  line L428 (35.2488, 47.5145) -> (38.7843, 43.9789)
  line L429 (38.7843, 51.05) -> (35.2488, 47.5145)
  line L430 (38.7843, 43.9789) -> (42.3198, 47.5145)
  line L431 (42.3198, 47.5145) -> (38.7843, 51.05)
  line L432 (31.645, 46.56) -> (-41.855, 46.56) construction
  line L433 (40.716, 46.56) -> (-32.784, 46.56) construction
  line L434 (26.1778, 47.5145) -> (29.7133, 43.9789)
  line L435 (29.7133, 51.05) -> (26.1778, 47.5145)
  line L436 (29.7133, 43.9789) -> (33.2488, 47.5145)
  line L437 (33.2488, 47.5145) -> (29.7133, 51.05)
  line L438 (22.574, 46.56) -> (-50.926, 46.56) construction
  line L439 (31.645, 46.56) -> (-41.855, 46.56) construction
  line L440 (17.1068, 47.5145) -> (20.6423, 43.9789)
  line L441 (20.6423, 51.05) -> (17.1068, 47.5145)
  line L442 (20.6423, 43.9789) -> (24.1778, 47.5145)
  line L443 (24.1778, 47.5145) -> (20.6423, 51.05)
  line L444 (13.503, 46.56) -> (-59.997, 46.56) construction
  line L445 (22.574, 46.56) -> (-50.926, 46.56) construction
  line L446 (8.0358, 47.5145) -> (11.5713, 43.9789)
  line L447 (11.5713, 51.05) -> (8.0358, 47.5145)
  line L448 (11.5713, 43.9789) -> (15.1068, 47.5145)
  line L449 (15.1068, 47.5145) -> (11.5713, 51.05)
  line L450 (67.929, 37.58) -> (-5.571, 37.58) construction
  line L451 (77, 37.58) -> (3.5, 37.58) construction
  line L452 (62.4618, 38.5345) -> (65.9973, 34.9989)
  line L453 (65.9973, 42.07) -> (62.4618, 38.5345)
  line L454 (65.9973, 34.9989) -> (69.5328, 38.5345)
  line L455 (69.5328, 38.5345) -> (65.9973, 42.07)
  line L456 (58.858, 37.58) -> (-14.642, 37.58) construction
  line L457 (67.929, 37.58) -> (-5.571, 37.58) construction
  line L458 (53.3908, 38.5345) -> (56.9263, 34.9989)
  line L459 (56.9263, 42.07) -> (53.3908, 38.5345)
  line L460 (56.9263, 34.9989) -> (60.4618, 38.5345)
  line L461 (60.4618, 38.5345) -> (56.9263, 42.07)
  line L462 (49.787, 37.58) -> (-23.713, 37.58) construction
  line L463 (58.858, 37.58) -> (-14.642, 37.58) construction
  line L464 (44.3198, 38.5345) -> (47.8553, 34.9989)
  line L465 (47.8553, 42.07) -> (44.3198, 38.5345)
  line L466 (47.8553, 34.9989) -> (51.3908, 38.5345)
  line L467 (51.3908, 38.5345) -> (47.8553, 42.07)
  line L468 (40.716, 37.58) -> (-32.784, 37.58) construction
  line L469 (49.787, 37.58) -> (-23.713, 37.58) construction
  line L470 (35.2488, 38.5345) -> (38.7843, 34.9989)
  line L471 (38.7843, 42.07) -> (35.2488, 38.5345)
  line L472 (38.7843, 34.9989) -> (42.3198, 38.5345)
  line L473 (42.3198, 38.5345) -> (38.7843, 42.07)
  line L474 (31.645, 37.58) -> (-41.855, 37.58) construction
  line L475 (40.716, 37.58) -> (-32.784, 37.58) construction
  line L476 (26.1778, 38.5345) -> (29.7133, 34.9989)
  line L477 (29.7133, 42.07) -> (26.1778, 38.5345)
  line L478 (29.7133, 34.9989) -> (33.2488, 38.5345)
  line L479 (33.2488, 38.5345) -> (29.7133, 42.07)
  line L480 (22.574, 37.58) -> (-50.926, 37.58) construction
  line L481 (31.645, 37.58) -> (-41.855, 37.58) construction
  line L482 (17.1068, 38.5345) -> (20.6423, 34.9989)
  line L483 (20.6423, 42.07) -> (17.1068, 38.5345)
  line L484 (20.6423, 34.9989) -> (24.1778, 38.5345)
  line L485 (24.1778, 38.5345) -> (20.6423, 42.07)
  line L486 (13.503, 37.58) -> (-59.997, 37.58) construction
  line L487 (22.574, 37.58) -> (-50.926, 37.58) construction
  line L488 (8.0358, 38.5345) -> (11.5713, 34.9989)
  line L489 (11.5713, 42.07) -> (8.0358, 38.5345)
  line L490 (11.5713, 34.9989) -> (15.1068, 38.5345)
  line L491 (15.1068, 38.5345) -> (11.5713, 42.07)
  line L492 (67.929, 28.6) -> (-5.571, 28.6) construction
  line L493 (77, 28.6) -> (3.5, 28.6) construction
  line L494 (62.4618, 29.5545) -> (65.9973, 26.0189)
  line L495 (65.9973, 33.09) -> (62.4618, 29.5545)
  line L496 (65.9973, 26.0189) -> (69.5328, 29.5545)
  line L497 (69.5328, 29.5545) -> (65.9973, 33.09)
  line L498 (58.858, 28.6) -> (-14.642, 28.6) construction
  line L499 (67.929, 28.6) -> (-5.571, 28.6) construction
  line L500 (53.3908, 29.5545) -> (56.9263, 26.0189)
  line L501 (56.9263, 33.09) -> (53.3908, 29.5545)
  line L502 (56.9263, 26.0189) -> (60.4618, 29.5545)
  line L503 (60.4618, 29.5545) -> (56.9263, 33.09)
  line L504 (49.787, 28.6) -> (-23.713, 28.6) construction
  line L505 (58.858, 28.6) -> (-14.642, 28.6) construction
  line L506 (44.3198, 29.5545) -> (47.8553, 26.0189)
  line L507 (47.8553, 33.09) -> (44.3198, 29.5545)
  line L508 (47.8553, 26.0189) -> (51.3908, 29.5545)
  line L509 (51.3908, 29.5545) -> (47.8553, 33.09)
  line L510 (40.716, 28.6) -> (-32.784, 28.6) construction
  line L511 (49.787, 28.6) -> (-23.713, 28.6) construction
  line L512 (35.2488, 29.5545) -> (38.7843, 26.0189)
  line L513 (38.7843, 33.09) -> (35.2488, 29.5545)
  line L514 (38.7843, 26.0189) -> (42.3198, 29.5545)
  line L515 (42.3198, 29.5545) -> (38.7843, 33.09)
  line L516 (31.645, 28.6) -> (-41.855, 28.6) construction
  line L517 (40.716, 28.6) -> (-32.784, 28.6) construction
  line L518 (26.1778, 29.5545) -> (29.7133, 26.0189)
  line L519 (29.7133, 33.09) -> (26.1778, 29.5545)
  line L520 (29.7133, 26.0189) -> (33.2488, 29.5545)
  line L521 (33.2488, 29.5545) -> (29.7133, 33.09)
  line L522 (22.574, 28.6) -> (-50.926, 28.6) construction
  line L523 (31.645, 28.6) -> (-41.855, 28.6) construction
  line L524 (17.1068, 29.5545) -> (20.6423, 26.0189)
  line L525 (20.6423, 33.09) -> (17.1068, 29.5545)
  line L526 (20.6423, 26.0189) -> (24.1778, 29.5545)
  line L527 (24.1778, 29.5545) -> (20.6423, 33.09)
  line L528 (13.503, 28.6) -> (-59.997, 28.6) construction
  line L529 (22.574, 28.6) -> (-50.926, 28.6) construction
  line L530 (8.0358, 29.5545) -> (11.5713, 26.0189)
  line L531 (11.5713, 33.09) -> (8.0358, 29.5545)
  line L532 (11.5713, 26.0189) -> (15.1068, 29.5545)
  line L533 (15.1068, 29.5545) -> (11.5713, 33.09)
  line L534 (67.929, 19.62) -> (-5.571, 19.62) construction
  line L535 (77, 19.62) -> (3.5, 19.62) construction
  line L536 (62.4618, 20.5745) -> (65.9973, 17.0389)
  line L537 (65.9973, 24.11) -> (62.4618, 20.5745)
  line L538 (65.9973, 17.0389) -> (69.5328, 20.5745)
  line L539 (69.5328, 20.5745) -> (65.9973, 24.11)
  line L540 (58.858, 19.62) -> (-14.642, 19.62) construction
  line L541 (67.929, 19.62) -> (-5.571, 19.62) construction
  line L542 (53.3908, 20.5745) -> (56.9263, 17.0389)
  line L543 (56.9263, 24.11) -> (53.3908, 20.5745)
  line L544 (56.9263, 17.0389) -> (60.4618, 20.5745)
  line L545 (60.4618, 20.5745) -> (56.9263, 24.11)
  line L546 (49.787, 19.62) -> (-23.713, 19.62) construction
  line L547 (58.858, 19.62) -> (-14.642, 19.62) construction
  line L548 (44.3198, 20.5745) -> (47.8553, 17.0389)
  line L549 (47.8553, 24.11) -> (44.3198, 20.5745)
  line L550 (47.8553, 17.0389) -> (51.3908, 20.5745)
  line L551 (51.3908, 20.5745) -> (47.8553, 24.11)
  line L552 (40.716, 19.62) -> (-32.784, 19.62) construction
  line L553 (49.787, 19.62) -> (-23.713, 19.62) construction
  line L554 (35.2488, 20.5745) -> (38.7843, 17.0389)
  line L555 (38.7843, 24.11) -> (35.2488, 20.5745)
  line L556 (38.7843, 17.0389) -> (42.3198, 20.5745)
  line L557 (42.3198, 20.5745) -> (38.7843, 24.11)
  line L558 (31.645, 19.62) -> (-41.855, 19.62) construction
  line L559 (40.716, 19.62) -> (-32.784, 19.62) construction
  line L560 (26.1778, 20.5745) -> (29.7133, 17.0389)
  line L561 (29.7133, 24.11) -> (26.1778, 20.5745)
  line L562 (29.7133, 17.0389) -> (33.2488, 20.5745)
  line L563 (33.2488, 20.5745) -> (29.7133, 24.11)
  line L564 (22.574, 19.62) -> (-50.926, 19.62) construction
  line L565 (31.645, 19.62) -> (-41.855, 19.62) construction
  line L566 (17.1068, 20.5745) -> (20.6423, 17.0389)
  line L567 (20.6423, 24.11) -> (17.1068, 20.5745)
  line L568 (20.6423, 17.0389) -> (24.1778, 20.5745)
  line L569 (24.1778, 20.5745) -> (20.6423, 24.11)
  line L570 (13.503, 19.62) -> (-59.997, 19.62) construction
  line L571 (22.574, 19.62) -> (-50.926, 19.62) construction
  line L572 (8.0358, 20.5745) -> (11.5713, 17.0389)
  line L573 (11.5713, 24.11) -> (8.0358, 20.5745)
  line L574 (11.5713, 17.0389) -> (15.1068, 20.5745)
  line L575 (15.1068, 20.5745) -> (11.5713, 24.11)
  line L576 (67.929, 10.64) -> (-5.571, 10.64) construction
  line L577 (77, 10.64) -> (3.5, 10.64) construction
  line L578 (62.4618, 11.5945) -> (65.9973, 8.0589)
  line L579 (65.9973, 15.13) -> (62.4618, 11.5945)
  line L580 (65.9973, 8.0589) -> (69.5328, 11.5945)
  line L581 (69.5328, 11.5945) -> (65.9973, 15.13)
  line L582 (58.858, 10.64) -> (-14.642, 10.64) construction
  line L583 (67.929, 10.64) -> (-5.571, 10.64) construction
  line L584 (53.3908, 11.5945) -> (56.9263, 8.0589)
  line L585 (56.9263, 15.13) -> (53.3908, 11.5945)
  line L586 (56.9263, 8.0589) -> (60.4618, 11.5945)
  line L587 (60.4618, 11.5945) -> (56.9263, 15.13)
  line L588 (49.787, 10.64) -> (-23.713, 10.64) construction
  line L589 (58.858, 10.64) -> (-14.642, 10.64) construction
  line L590 (44.3198, 11.5945) -> (47.8553, 8.0589)
  line L591 (47.8553, 15.13) -> (44.3198, 11.5945)
  line L592 (47.8553, 8.0589) -> (51.3908, 11.5945)
  line L593 (51.3908, 11.5945) -> (47.8553, 15.13)
  line L594 (40.716, 10.64) -> (-32.784, 10.64) construction
  line L595 (49.787, 10.64) -> (-23.713, 10.64) construction
  line L596 (35.2488, 11.5945) -> (38.7843, 8.0589)
  line L597 (38.7843, 15.13) -> (35.2488, 11.5945)
  line L598 (38.7843, 8.0589) -> (42.3198, 11.5945)
  line L599 (42.3198, 11.5945) -> (38.7843, 15.13)
  line L600 (31.645, 10.64) -> (-41.855, 10.64) construction
  line L601 (40.716, 10.64) -> (-32.784, 10.64) construction
  line L602 (26.1778, 11.5945) -> (29.7133, 8.0589)
  line L603 (29.7133, 15.13) -> (26.1778, 11.5945)
  line L604 (29.7133, 8.0589) -> (33.2488, 11.5945)
  line L605 (33.2488, 11.5945) -> (29.7133, 15.13)
  line L606 (22.574, 10.64) -> (-50.926, 10.64) construction
  line L607 (31.645, 10.64) -> (-41.855, 10.64) construction
  line L608 (17.1068, 11.5945) -> (20.6423, 8.0589)
  line L609 (20.6423, 15.13) -> (17.1068, 11.5945)
  line L610 (20.6423, 8.0589) -> (24.1778, 11.5945)
  line L611 (24.1778, 11.5945) -> (20.6423, 15.13)
  line L612 (13.503, 10.64) -> (-59.997, 10.64) construction
  line L613 (22.574, 10.64) -> (-50.926, 10.64) construction
  line L614 (8.0358, 11.5945) -> (11.5713, 8.0589)
  line L615 (11.5713, 15.13) -> (8.0358, 11.5945)
  line L616 (11.5713, 8.0589) -> (15.1068, 11.5945)
  line L617 (15.1068, 11.5945) -> (11.5713, 15.13)
  point P0 (38.5, 0)
  dimension "d58" = 5
  dimension "d59" = 5
  dimension "d60" = 0
  dimension "d61" = 2.932
  dimension "d62" = 3.5
  dimension "d63" = 7.0711
  dimension "d66" = 9.071
  dimension "d69" = 8.98
  dimension "d72" = 5
  dimension "d73" = 5
  dimension "d74" = 1.3818
  dimension "d75" = 1.3822
  dimension "d76" = 1.3818
  dimension "d77" = 1.3822
  dimension "d80" = 9.071
  dimension "d83" = 8.98
  constraints: 1228 end point, 5 parallel, 3 horizontal, 3 perpendicular, 2 vertical, 1365 other
  measures "d58" distance between parallel lines of L8 L6
  measures "d59" distance between parallel lines of L7 L9
  measures "d60" distance from line of L1 L6.end
  measures "d61" distance from line of L10 L7.end
  measures "d62" distance from line of L0 L6.end
  measures "d63" distance of L6.start L7.end
  measures "d66" distance of L8.end L11.start
  measures "d69" distance of L8.end L46.start
  measures "d72" distance between parallel lines of L329 L327
  measures "d73" distance between parallel lines of L326 L328
  measures "d74" distance between parallel lines of L327 L9
  measures "d75" distance between parallel lines of L52 L329
  measures "d76" distance between parallel lines of L50 L326
  measures "d77" distance between parallel lines of L13 L328
  measures "d80" distance of L54.start L330.start
  measures "d83" distance of L54.start L366.start
extrude "Swiss-ified" cut sketch "Swiss Holes Sketch" against normal through all